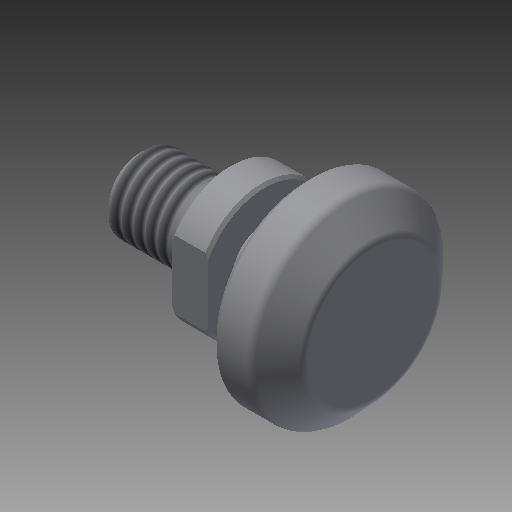
# Autodesk Inventor part: MayTec 1.67.42E3M8_Slot roller E3
Saved by Autodesk Inventor 2018 (Build 220112000, 112)
## iProperties
Category: PARTsolutions
Company: MAYTEC
Created: 2012-11-14
Part Number: MayTec 1.67.42E3M8_Slot roller E3
Catalog Web Link: www.cadenas.de
Description: 1.67.42E-Slot roller
Vendor: MAYTEC
Document SubType Name: Modeling
Designer: PARTuser1
Manufacturer: MAYTEC
Density: 1 g/cm^3
Material: Generic
Appearance: RGB(175.94999939203154,175.94999939203154,175.94999939203154)
PSOL_IDENT_0: {\\10.0.0.242\data_v9\23d-libs\maytec\maytec_3d\anbauzubehoer\laufrollen\laufrolle.prj},210 {VTYP=3D
PSOL_IDENT_1: },{NB=MayTec 1.67.42E3M8_Slot roller E3},{LINA=MayTec 1.67.42E3M8_Slot roller E3},{NN=1.67.42E},{DAT
PSOL_IDENT_2: E=14.09.2010 08:31:54},{GEOMDATE=28.01.2010 00:00:00},{VERSION=},{LINEID=20},{LINESUBID=-1},{WBVAR=}
PSOL_IDENT_3: {NB=MayTec 1.67.42E3M8_Slot roller E3},{LINA=MayTec 1.67.42E3M8_Slot roller E3},{KT=DUMMY},{PARTNR
PSOL_IDENT_4: =1.67.42E3M8},{DESCRIPTION=Laufrolle E3},{XTRANS=Slot roller E3},{A=4.45}
CNS_NT: Slot roller
CNS_NB: MayTec 1.67.42E3M8_Slot roller E3
CNS_NBSYN: MayTec $PARTNR._$XTRANS.
CNS_LINA: MayTec 1.67.42E3M8_Slot roller E3
CNS_PARTNR: 1.67.42E3M8
CNS_DESCRIPTION: Slot roller E3
CNS_XTRANS: Slot roller E3
CNS_A: 4.45
SUPPLIER: MAYTEC
ARTICLENO: MayTec 1.67.42E3M8_Slot roller E3
BOMINFO: MayTec 1.67.42E3M8_Slot roller E3
CREATOR: CADENAS GmbH
Title: MayTec 1.67.42E3M8_Slot roller E3
Author: Cadenas PARTsolutions
Comments: Slot roller
Autodesk Inventor part; units mm, degrees
sketch "Skizze_1" plane through (0, 0, 0) normal (0, 0, 1) x (1, 0, 0)
  line L0 (24.75, 0) -> (0, 0)
  line L1 (0, 0) -> (0, 3.233)
  line L2 (0, 3.233) -> (0.767, 4)
  line L3 (0.767, 4) -> (7, 4)
  line L4 (7, 4) -> (8, 3.35)
  line L5 (8, 3.35) -> (9.5, 3.35)
  line L6 (9.5, 3.35) -> (9.5, 6.7172)
  line L7 (9.5, 6.7172) -> (9.7828, 7)
  line L8 (9.7828, 7) -> (13.0172, 7)
  line L9 (13.0172, 7) -> (13.3, 6.7172)
  line L10 (13.3, 6.7172) -> (13.3, 3.5)
  line L11 (13.3, 3.5) -> (17.75, 3.5)
  line L12 (17.75, 3.5) -> (17.75, 9.5429)
  line L13 (17.75, 9.5429) -> (18.4571, 10.25)
  line L14 (18.4571, 10.25) -> (21.5622, 10.25)
  arc A0 (22.297, 9.9283) -> (21.5622, 10.25) centre (21.5622, 9.25) ccw
  line L15 (22.297, 9.9283) -> (24.4848, 7.5581)
  arc A1 (24.75, 6.8798) -> (24.4848, 7.5581) centre (23.75, 6.8798) ccw
  line L16 (24.75, 6.8798) -> (24.75, 0)
  line L17 (24.75, 0) -> (0, 0)
  constraints: 36 end point, 4 point on circle, 2 centre point
revolve "Revolution1" add sketch "Skizze_1" angle 360 about axis through (24.75, 0, 0) along (1, 0, 0)
thread "Thread1" size "M8x1.25" class "6g" standard "ISO Metric profile" full length
sketch "Skizze_2" plane through (0, 0, 0) normal (0, 1, 0) x (-1, 0, 0)
  line L0 (-6, 6) -> (-6, 14)
  line L1 (-6, 14) -> (-14, 14)
  line L2 (-14, 14) -> (-14, 6)
  line L3 (-14, 6) -> (-6, 6)
  constraints: 8 end point
extrude "Extrusion1" cut sketch "Skizze_2" along normal mid plane 10
sketch "Skizze_3" plane through (0, 0, 0) normal (0, 1, 0) x (-1, 0, 0)
  line L0 (-6, -14) -> (-6, -6)
  line L1 (-6, -6) -> (-14, -6)
  line L2 (-14, -6) -> (-14, -14)
  line L3 (-14, -14) -> (-6, -14)
  constraints: 8 end point
extrude "Extrusion2" cut sketch "Skizze_3" along normal mid plane 10
ref_plane "side_1_XY" through (9.5, 0, 0) normal (-1, 0, 0) x (0, 0, -1)
ref_plane "side_1_YZ" through (9.5, 0, 0) normal (0, 0, -1) x (0, -1, 0)
ref_plane "side_1_ZX" through (9.5, 0, 0) normal (0, -1, 0) x (-1, 0, 0)
ref_plane "side_2_XY" through (14.6, 0, 0) normal (1, 0, 0) x (0, 0, -1)
ref_plane "side_2_YZ" through (14.6, 0, 0) normal (0, 0, -1) x (0, 1, 0)
ref_plane "side_2_ZX" through (14.6, 0, 0) normal (0, 1, 0) x (1, 0, 0)
body "Solid1"
